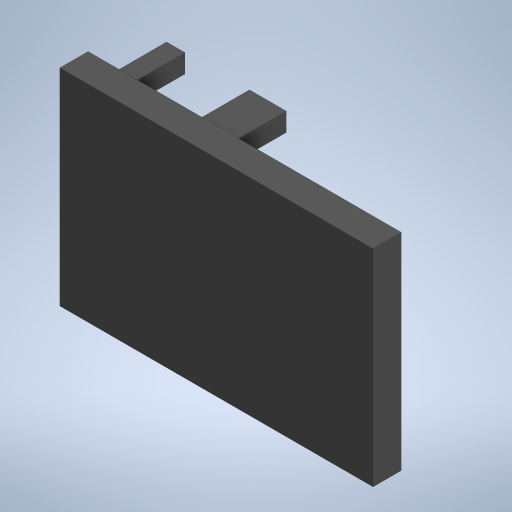
# Autodesk Inventor part: lcd 디스플레이
Saved by Autodesk Inventor 2023.1 (Build 271208000, 208)
## iProperties
Created: 2022-06-05
Part Number: lcd 디스플레이
Material: 일반
Document SubType Name: Modeling
Designer: fly01
Density: 1 g/cm^3
Appearance: 기본값
Author: fly01
Autodesk Inventor part; units mm, degrees
ref_plane "YZ Plane" through (0, 0, 0) normal (1, 0, 0) x (0, 1, 0)
ref_plane "XZ Plane" through (0, 0, 0) normal (0, 1, 0) x (-1, 0, 0)
ref_plane "XY Plane" through (0, 0, 0) normal (0, 0, 1) x (1, 0, 0)
sketch "스케치2" plane through (0, 0, 0) normal (0, 0, 1) x (1, 0, 0)
  line L0 (-42.5, 28) -> (42.5, 28)
  line L1 (42.5, 28) -> (42.5, -28)
  line L2 (42.5, -28) -> (-42.5, -28)
  line L3 (-42.5, -28) -> (-42.5, 28)
  line L4 (-42.5, 28) -> (42.5, -28) construction
  line L5 (42.5, 28) -> (-42.5, -28) construction
  point P0 (0, 0)
  dimension "d6" = 85
  dimension "d7" = 56
  constraints: 12 end point, 2 midpoint, 2 parallel, 1 horizontal, 1 perpendicular
  measures "d6" distance of L1.end L2.end
  measures "d7" distance of L0.end L1.end
extrude "돌출2" add sketch "스케치2" along normal blind 7.65
sketch "스케치4" plane through (0, 0, 0) normal (0, 0, -1) x (-1, 0, 0)
  line L0 (30, 27.091) -> (35, 27.091)
  line L1 (35, 27.091) -> (35, 22.091)
  line L2 (35, 22.091) -> (30, 22.091)
  line L3 (30, 22.091) -> (30, 27.091)
  line L4 (30, 27.091) -> (35, 22.091) construction
  line L5 (35, 27.091) -> (30, 22.091) construction
  line L6 (-42.5, 28) -> (42.5, 28) projected
  line L7 (-42.5, -28) -> (-42.5, 28) projected
  line L8 (30.95, 25.541) -> (31.55, 25.541)
  line L9 (31.55, 25.541) -> (31.55, 26.141)
  line L10 (31.55, 26.141) -> (30.95, 26.141)
  line L11 (30.95, 26.141) -> (30.95, 25.541)
  line L12 (30.95, 25.541) -> (31.55, 26.141) construction
  line L13 (31.55, 25.541) -> (30.95, 26.141) construction
  line L14 (32.5, 24.591) -> (32.5, 25.0687)
  line L15 (32.5, 24.591) -> (32.0223, 24.591)
  line L16 (34.05, 25.541) -> (33.45, 25.541)
  line L17 (33.45, 25.541) -> (33.45, 26.141)
  line L18 (33.45, 26.141) -> (34.05, 26.141)
  line L19 (34.05, 26.141) -> (34.05, 25.541)
  line L20 (34.05, 25.541) -> (33.45, 26.141) construction
  line L21 (33.45, 25.541) -> (34.05, 26.141) construction
  line L22 (30.95, 23.641) -> (31.55, 23.641)
  line L23 (31.55, 23.641) -> (31.55, 23.041)
  line L24 (31.55, 23.041) -> (30.95, 23.041)
  line L25 (30.95, 23.041) -> (30.95, 23.641)
  line L26 (30.95, 23.641) -> (31.55, 23.041) construction
  line L27 (31.55, 23.641) -> (30.95, 23.041) construction
  line L28 (34.05, 23.641) -> (33.45, 23.641)
  line L29 (33.45, 23.641) -> (33.45, 23.041)
  line L30 (33.45, 23.041) -> (34.05, 23.041)
  line L31 (34.05, 23.041) -> (34.05, 23.641)
  line L32 (34.05, 23.641) -> (33.45, 23.041) construction
  line L33 (33.45, 23.641) -> (34.05, 23.041) construction
  line L34 (42.5, 28) -> (42.5, -28) projected
  line L35 (12.5, 22.091) -> (2.5, 22.091)
  line L36 (2.5, 22.091) -> (2.5, 27.091)
  line L37 (2.5, 27.091) -> (12.5, 27.091)
  line L38 (12.5, 27.091) -> (12.5, 22.091)
  line L39 (12.5, 22.091) -> (2.5, 27.091) construction
  line L40 (2.5, 22.091) -> (12.5, 27.091) construction
  line L41 (11.55, 23.641) -> (10.95, 23.641)
  line L42 (10.95, 23.641) -> (10.95, 23.041)
  line L43 (10.95, 23.041) -> (11.55, 23.041)
  line L44 (11.55, 23.041) -> (11.55, 23.641)
  line L45 (11.55, 23.641) -> (10.95, 23.041) construction
  line L46 (10.95, 23.641) -> (11.55, 23.041) construction
  line L47 (11.55, 25.541) -> (11.55, 26.141)
  line L48 (10.95, 26.141) -> (10.95, 25.541)
  line L49 (10.95, 25.541) -> (11.55, 25.541)
  line L50 (11.55, 26.141) -> (10.95, 26.141)
  line L51 (11.55, 26.141) -> (10.95, 25.541) construction
  line L52 (10.95, 26.141) -> (11.55, 25.541) construction
  line L53 (9.05, 23.041) -> (9.05, 23.641)
  line L54 (8.45, 23.641) -> (8.45, 23.041)
  line L55 (8.45, 23.041) -> (9.05, 23.041)
  line L56 (9.05, 23.641) -> (8.45, 23.641)
  line L57 (9.05, 23.641) -> (8.45, 23.041) construction
  line L58 (8.45, 23.641) -> (9.05, 23.041) construction
  line L59 (9.05, 25.541) -> (9.05, 26.141)
  line L60 (8.45, 26.141) -> (8.45, 25.541)
  line L61 (8.45, 25.541) -> (9.05, 25.541)
  line L62 (9.05, 26.141) -> (8.45, 26.141)
  line L63 (9.05, 26.141) -> (8.45, 25.541) construction
  line L64 (8.45, 26.141) -> (9.05, 25.541) construction
  line L65 (6.55, 23.041) -> (6.55, 23.641)
  line L66 (5.95, 23.641) -> (5.95, 23.041)
  line L67 (5.95, 23.041) -> (6.55, 23.041)
  line L68 (6.55, 23.641) -> (5.95, 23.641)
  line L69 (6.55, 23.641) -> (5.95, 23.041) construction
  line L70 (5.95, 23.641) -> (6.55, 23.041) construction
  line L71 (6.55, 25.541) -> (6.55, 26.141)
  line L72 (5.95, 26.141) -> (5.95, 25.541)
  line L73 (5.95, 25.541) -> (6.55, 25.541)
  line L74 (6.55, 26.141) -> (5.95, 26.141)
  line L75 (6.55, 26.141) -> (5.95, 25.541) construction
  line L76 (5.95, 26.141) -> (6.55, 25.541) construction
  line L77 (4.05, 23.041) -> (4.05, 23.641)
  line L78 (3.45, 23.641) -> (3.45, 23.041)
  line L79 (3.45, 23.041) -> (4.05, 23.041)
  line L80 (4.05, 23.641) -> (3.45, 23.641)
  line L81 (4.05, 23.641) -> (3.45, 23.041) construction
  line L82 (3.45, 23.641) -> (4.05, 23.041) construction
  line L83 (4.05, 25.541) -> (4.05, 26.141)
  line L84 (3.45, 26.141) -> (3.45, 25.541)
  line L85 (3.45, 25.541) -> (4.05, 25.541)
  line L86 (4.05, 26.141) -> (3.45, 26.141)
  line L87 (4.05, 26.141) -> (3.45, 25.541) construction
  line L88 (3.45, 26.141) -> (4.05, 25.541) construction
  point P0 (0, 0)
  point P1 (31.25, 25.841)
  point P2 (33.75, 25.841)
  point P3 (31.25, 23.341)
  point P4 (33.75, 23.341)
  point P5 (7.5, 24.591)
  point P6 (11.25, 23.341)
  point P7 (11.25, 25.841)
  point P8 (8.75, 23.341)
  point P9 (8.75, 25.841)
  point P10 (6.25, 23.341)
  point P11 (6.25, 25.841)
  point P12 (3.75, 23.341)
  point P13 (3.75, 25.841)
  dimension "d12" = 5
  dimension "d13" = 5
  dimension "d14" = 0.6
  dimension "d15" = 0.6
  dimension "d18" = 1.25
  dimension "d19" = 7.5
  dimension "d20" = 0.909
  dimension "d21" = 5
  dimension "d22" = 10
  dimension "d23" = 17.5
  dimension "d24" = 0.909
  dimension "d25" = 0.6
  dimension "d26" = 0.6
  dimension "d27" = 1.25
  dimension "d28" = 1.25
  dimension "d31" = 2.5
  dimension "d34" = 2.5
  constraints: 172 end point, 15 symmetric about line, 8 midpoint, 8 parallel, 6 horizontal, 4 perpendicular, 2 vertical, 1 point on line, 77 other
  measures "d12" distance of L2.end L0.start
  measures "d13" distance of L0.start L0.end
  measures "d14" distance of L10.end L9.end
  measures "d15" distance of L9.end L8.end
  measures "d18" distance from line of L14 point (31.25, 25.841)
  measures "d19" distance between parallel lines of L34 L1
  measures "d20" distance between parallel lines of L6 L0
  measures "d21" distance of L37.end L35.start
  measures "d22" distance of L35.start L35.end
  measures "d23" distance between parallel lines of L3 L38
  measures "d24" distance between parallel lines of L6 L37
  measures "d25" distance of L43.end L42.end
  measures "d26" distance of L42.end L41.end
  measures "d27" distance from line of L38 point (11.25, 23.341)
  measures "d28" distance from line of L35 point (11.25, 23.341)
  measures "d31" distance of L43.end L47.start
  measures "d34" distance of L43.end L53.start
extrude "돌출3" add sketch "스케치4" along normal blind 13.8
sketch "스케치5" plane through (-42.5, -28, 0) normal (0, -1, 0) x (1, 0, 0)
  line L0 (85, 0) -> (0, 0) projected
  line L1 (24, 0) -> (39.15, 0)
  line L2 (39.15, 0) -> (39.15, -6.2)
  line L3 (39.15, -6.2) -> (24, -6.2)
  line L4 (24, -6.2) -> (24, 0)
  line L5 (0, 0) -> (0, 7.65) projected
  line L6 (24, -2.9) -> (24.5, -2.9)
  line L7 (26.5, -0.9) -> (26.5, -0.9)
  line L8 (27, -0.4) -> (36.05, -0.4)
  line L9 (36.55, 0) -> (36.55, -13.8) construction
  line L10 (36.55, -0.9) -> (36.55, -0.9)
  line L11 (38.55, -2.9) -> (39.05, -2.9)
  line L12 (39.05, 0) -> (39.05, -13.8) projected
  arc A0 (24.5, -2.9) -> (26.5, -0.9) centre (24.5, -0.9) ccw
  arc A1 (36.55, -0.9) -> (38.55, -2.9) centre (38.55, -0.9) ccw
  arc A2 (27, -0.4) -> (26.5, -0.9) centre (27, -0.9) ccw
  arc A3 (36.55, -0.9) -> (36.05, -0.4) centre (36.05, -0.9) ccw
  line L13 (24.5, -2.9) -> (24.5, 0.0781)
  line L14 (38.55, -2.9) -> (38.55, 0)
  point P0 (42.5, 0)
  point P1 (26.5, -2.9)
  point P2 (26.5, -0.4)
  point P3 (36.55, -2.9)
  point P4 (36.55, -0.9)
  point P5 (26.5, -0.9)
  point P6 (24.5, 0)
  point P7 (39.05, -6.2)
  dimension "d37" = 24
  dimension "d38" = 15.15
  dimension "d39" = 6.2
  dimension "d40" = 2.5
  dimension "d41" = 2.5
  dimension "d42" = 3.3
  dimension "d43" = 2.5
  dimension "d44" = 2
  dimension "d45" = 0.5
  constraints: 22 end point, 12 point on line, 8 point on circle, 8 tangent, 6 perpendicular, 4 centre point, 2 equal radius, 2 horizontal, 2 parallel
  measures "d37" distance between parallel lines of L5 L4
  measures "d38" distance of L2.end L3.end
  measures "d39" distance of L3.end L1.start
  measures "d40" distance of point (26.5, -2.9) point (26.5, -0.4)
  measures "d41" distance of L6.start point (26.5, -2.9)
  measures "d42" distance between parallel lines of L3 L6
  measures "d43" distance of point (36.55, -2.9) L11.end
  measures "d44" radius of A0
  measures "d45" radius of A2
extrude "돌출4" add sketch "스케치5" against normal blind 12.1 contours L12 L11 L14 L0 | L12 L3 L4 L6 A0 A2 L8 A3 A1 L11 | L13 L6 L4 L0
fillet "모깎기1" radius 1 2 edges at (-18.5, -21.95, -6.2) (-3.45, -21.95, -6.2)
extrude "돌출5" cut sketch "스케치5" against normal blind 1 contours L12 L11 L14 L0 | L13 L6 L4 L0
sketch "스케치6" plane through (-15.5, -28, -0.4) normal (0, -1, 0) x (1, 0, 0)
  line L0 (12.05, -2.5) -> (11.55, -2.5) projected
  arc A0 (9.55, -0.5) -> (11.55, -2.5) centre (11.55, -0.5) ccw projected
  arc A1 (9.55, -0.5) -> (9.05, 0) centre (9.05, -0.5) ccw projected
  line L1 (9.05, 0) -> (0, 0) projected
  arc A2 (0, 0) -> (-0.5, -0.5) centre (0, -0.5) ccw projected
  arc A3 (-2.5, -2.5) -> (-0.5, -0.5) centre (-2.5, -0.5) ccw projected
  line L2 (-2.5, -2.5) -> (-3, -2.5) projected
  line L3 (-3, -2.5) -> (-3, -4.8) projected
  arc A4 (-3, -4.8) -> (-2, -5.8) centre (-2, -4.8) ccw projected
  line L4 (-2, -5.8) -> (11.05, -5.8) projected
  arc A5 (11.05, -5.8) -> (12.05, -4.8) centre (11.05, -4.8) ccw projected
  line L5 (12.05, -4.8) -> (12.05, -2.5) projected
  line L6 (-2.5, -4.8) -> (-2.5, -3)
  line L7 (-2.5, -3) -> (-2.5, -3)
  arc A6 (-2.5, -3) -> (0, -0.5) centre (-2.5, -0.5) ccw
  line L8 (0, -0.5) -> (9.05, -0.5)
  arc A7 (9.05, -0.5) -> (11.55, -3) centre (11.55, -0.5) ccw
  line L9 (11.55, -3) -> (11.55, -3)
  line L10 (11.55, -3) -> (11.55, -4.8)
  arc A8 (11.05, -5.3) -> (11.55, -4.8) centre (11.05, -4.8) ccw
  line L11 (11.05, -5.3) -> (-2, -5.3)
  arc A9 (-2.5, -4.8) -> (-2, -5.3) centre (-2, -4.8) ccw
  point P0 (15.5, 0.4)
  point P1 (11.55, -3)
  point P2 (9.05, -0.5)
  point P3 (0, -0.5)
  point P4 (-2.5, -3)
  dimension "d51" = 0.5
  constraints: 12 end point, 8 point on circle, 4 centre point, 19 other
  measures "d51" distance between parallel lines of L3 L6
extrude "돌출6" cut sketch "스케치6" against normal blind 11.5 contours L6 A6 L8 A7 L10 A8 L11 A9
sketch "스케치7" plane through (-15.5, -28, -0.4) normal (0, -1, 0) x (1, 0, 0)
  arc A0 (9.05, -0.5) -> (11.55, -3) centre (11.55, -0.5) ccw projected
  line L0 (11.55, -3) -> (11.55, -4.8) projected
  arc A1 (11.05, -5.3) -> (11.55, -4.8) centre (11.05, -4.8) ccw projected
  line L1 (11.05, -5.3) -> (-2, -5.3) projected
  arc A2 (-2.5, -4.8) -> (-2, -5.3) centre (-2, -4.8) ccw projected
  line L2 (-2.5, -4.8) -> (-2.5, -3) projected
  arc A3 (-2.5, -3) -> (0, -0.5) centre (-2.5, -0.5) ccw projected
  line L3 (0, -0.5) -> (9.05, -0.5) projected
  line L4 (12.05, -2.5) -> (11.55, -2.5) projected
  arc A4 (9.55, -0.5) -> (11.55, -2.5) centre (11.55, -0.5) ccw projected
  arc A5 (9.55, -0.5) -> (9.05, 0) centre (9.05, -0.5) ccw projected
  line L5 (9.05, 0) -> (0, 0) projected
  arc A6 (0, 0) -> (-0.5, -0.5) centre (0, -0.5) ccw projected
  arc A7 (-2.5, -2.5) -> (-0.5, -0.5) centre (-2.5, -0.5) ccw projected
  line L6 (-2.5, -2.5) -> (-3, -2.5) projected
  line L7 (-3, -2.5) -> (-3, -4.8) projected
  arc A8 (-3, -4.8) -> (-2, -5.8) centre (-2, -4.8) ccw projected
  line L8 (-2, -5.8) -> (11.05, -5.8) projected
  arc A9 (11.05, -5.8) -> (12.05, -4.8) centre (11.05, -4.8) ccw projected
  line L9 (12.05, -4.8) -> (12.05, -2.5) projected
  point P0 (15.5, 0.4)
extrude "돌출7" add sketch "스케치7" along normal blind 0.7
